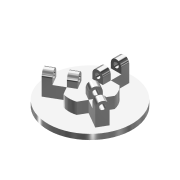
# Autodesk Inventor part: Base_Dedao
Saved by Autodesk Inventor 2020 (Build 240168000, 168)
## iProperties
Created: 2021-04-01
Part Number: Base_Dedao
Material: Generic
Document SubType Name: Modeling
Designer: deox
Density: 1 g/cm^3
Appearance: Chrome - Polished
Author: deox
Autodesk Inventor part; units mm, degrees
ref_plane "YZ Plane" through (0, 0, 0) normal (1, 0, 0) x (0, 1, 0)
ref_plane "XZ Plane" through (0, 0, 0) normal (0, 1, 0) x (-1, 0, 0)
ref_plane "XY Plane" through (0, 0, 0) normal (0, 0, 1) x (1, 0, 0)
sketch "Sketch1" plane through (0, 0, 0) normal (0, 1, 0) x (-1, 0, 0)
  circle A0 centre (0, 0) radius 11
  dimension "d0" = 22
  constraints: 1 centre point, 1 coincident
  measures "d0" diameter of A0
extrude "Extrusion1" add sketch "Sketch1" along normal blind 1.4
sketch "Sketch2" plane through (0, 1.4, 0) normal (0, 1, 0) x (1, 0, 0)
  line L0 (-11.1515, 11.0791) -> (11.8145, 11.0791) construction
  line L1 (11.8145, 11.0791) -> (11.8145, -11.3383) construction
  line L2 (11.8145, -11.3383) -> (-11.1515, -11.3383) construction
  line L3 (-11.1515, -11.3383) -> (-11.1515, 11.0791) construction
  circle A0 centre (0, 0) radius 11 projected
  circle A1 centre (0, 0) radius 11 projected
  line L4 (0, 0) -> (0, 2.0078)
  line L5 (0, 2.0078) -> (1.375, 2.0078)
  line L6 (1.375, 2.0078) -> (1.375, 4.0678)
  line L7 (1.375, 4.0678) -> (0, 4.0678)
  line L8 (1.375, 4.0678) -> (1.375, 6.8478)
  line L9 (1.375, 6.8478) -> (1.375, 8.9078)
  line L10 (1.375, 8.9078) -> (-1.375, 8.9078)
  line L11 (-1.375, 8.9078) -> (-1.375, 2.0078)
  line L12 (-1.375, 2.0078) -> (0, 2.0078)
  line L13 (1.375, 4.1034) -> (3.6499, 4.1034)
  line L14 (0, 0) -> (13.4051, 0) construction
  line L15 (4.2411, -0.8609) -> (5.3786, 1.1092)
  arc A2 (5.3786, 1.1092) -> (3.6499, 4.1034) centre (-0.1977, -0.1141) ccw
  line L16 (0, 0) -> (4.7463, 2.7403)
  line L17 (-1.7388, -1.0039) -> (-2.4263, 0.1869)
  line L18 (-2.4263, 0.1869) -> (-4.2104, -0.8431)
  line L19 (-4.2104, -0.8431) -> (-6.6179, -2.2331)
  line L20 (-1.0513, -2.1947) -> (-1.7388, -1.0039)
  line L21 (-6.6179, -2.2331) -> (-8.4019, -3.2631)
  line L22 (-7.0269, -5.6447) -> (-1.0513, -2.1947)
  line L23 (-8.4019, -3.2631) -> (-7.0269, -5.6447)
  line L24 (-4.2104, -0.8431) -> (-3.5229, -2.0339)
  line L25 (-4.2411, -0.8609) -> (-5.3786, 1.1092)
  line L26 (0, 0) -> (-1.7388, -1.0039)
  arc A3 (-3.6499, 4.1034) -> (-5.3786, 1.1092) centre (0.1977, -0.1141) ccw
  line L27 (0, 0) -> (-4.7463, 2.7403)
  line L28 (-1.375, 4.1034) -> (-3.6499, 4.1034)
  line L29 (1.7388, -1.0039) -> (1.0513, -2.1947)
  line L30 (1.0513, -2.1947) -> (2.8354, -3.2247)
  line L31 (2.8354, -3.2247) -> (5.2429, -4.6147)
  line L32 (2.4263, 0.1869) -> (1.7388, -1.0039)
  line L33 (5.2429, -4.6147) -> (7.0269, -5.6447)
  line L34 (8.4019, -3.2631) -> (2.4263, 0.1869)
  line L35 (7.0269, -5.6447) -> (8.4019, -3.2631)
  line L36 (2.8354, -3.2247) -> (3.5229, -2.0339)
  line L37 (2.8661, -3.2425) -> (1.7287, -5.2126)
  line L38 (0, 0) -> (1.7388, -1.0039)
  arc A4 (-1.7287, -5.2126) -> (1.7287, -5.2126) centre (0, 0.2283) ccw
  line L39 (0, 0) -> (0, -5.4806)
  line L40 (-2.8661, -3.2425) -> (-1.7287, -5.2126)
  dimension "d38" = 1.375
  dimension "d39" = 2.06
  dimension "d40" = 2.78
  dimension "d41" = 2.06
  dimension "d42" = 2.75
  dimension "d49" = 360
  dimension "d56" = 2.0078
  constraints: 74 end point, 9 point on circle, 9 point on line, 6 perpendicular, 3 centre point, 2 coincident, 2 horizontal, 2 vertical, 91 other
  measures "d38" distance of L4.end L5.end
  measures "d39" distance of L5.end L6.end
  measures "d40" distance of L6.end L8.end
  measures "d41" distance of L8.end L9.end
  measures "d42" distance of L9.end L10.end
  measures "d56" distance of L4.start L4.end
extrude "Extrusion2" add sketch "Sketch2" along normal blind 3 contours L27 A3 L28 L11 L12 L4 | L4 L5 L6 L8 L13 A2 L16 | L39 A4 L40 L22 L20 L26 | L26 L17 L18 L19 L25 A3 L27 | L16 A2 L15 L34 L32 L38 | L38 L29 L30 L31 L37 A4 L39 | L12 L11 L10 L9 L8 L6 L5 | L20 L22 L23 L21 L19 L18 L17 | L32 L34 L35 L33 L31 L30 L29
sketch "Sketch3" plane through (0, 4.4, 0) normal (0, 1, 0) x (1, 0, 0)
  line L0 (0, 0) -> (0, 2.0078)
  line L1 (0, 2.0078) -> (1.375, 2.0078)
  line L2 (1.375, 2.0078) -> (1.375, 4.0678)
  line L3 (1.375, 4.0678) -> (0, 4.0678)
  line L4 (0, 2.0078) -> (0, 4.0678)
  line L5 (1.375, 4.1034) -> (1.375, 8.9078) projected
  line L6 (1.375, 8.9078) -> (1.375, 6.8478)
  line L7 (1.375, 6.8478) -> (-1.375, 6.8478)
  line L8 (-1.375, 4.1034) -> (-1.375, 8.9078) projected
  line L9 (1.375, 8.9078) -> (-1.375, 8.9078) projected
  line L10 (-1.375, 6.8478) -> (-1.375, 8.9078)
  line L11 (-1.375, 8.9078) -> (1.375, 8.9078)
  line L12 (0, 2.0078) -> (-1.375, 2.0078)
  line L13 (-1.375, 2.0078) -> (-1.375, 4.0678)
  line L14 (-1.375, 4.0678) -> (0, 4.0678)
  line L15 (-1.7388, -1.0039) -> (-2.4263, 0.1869)
  line L16 (-2.4263, 0.1869) -> (-4.2104, -0.8431)
  line L17 (-4.2104, -0.8431) -> (-3.5229, -2.0339)
  line L18 (-1.7388, -1.0039) -> (-3.5229, -2.0339)
  line L19 (-1.7388, -1.0039) -> (-1.0513, -2.1947)
  line L20 (-1.0513, -2.1947) -> (-2.8354, -3.2247)
  line L21 (-2.8354, -3.2247) -> (-3.5229, -2.0339)
  line L22 (-8.4019, -3.2631) -> (-6.6179, -2.2331)
  line L23 (-6.6179, -2.2331) -> (-5.2429, -4.6147)
  line L24 (-5.2429, -4.6147) -> (-7.0269, -5.6447)
  line L25 (-7.0269, -5.6447) -> (-8.4019, -3.2631)
  line L26 (1.7388, -1.0039) -> (1.0513, -2.1947)
  line L27 (1.0513, -2.1947) -> (2.8354, -3.2247)
  line L28 (2.8354, -3.2247) -> (3.5229, -2.0339)
  line L29 (1.7388, -1.0039) -> (3.5229, -2.0339)
  line L30 (1.7388, -1.0039) -> (2.4263, 0.1869)
  line L31 (2.4263, 0.1869) -> (4.2104, -0.8431)
  line L32 (4.2104, -0.8431) -> (3.5229, -2.0339)
  line L33 (7.0269, -5.6447) -> (5.2429, -4.6147)
  line L34 (5.2429, -4.6147) -> (6.6179, -2.2331)
  line L35 (6.6179, -2.2331) -> (8.4019, -3.2631)
  line L36 (8.4019, -3.2631) -> (7.0269, -5.6447)
  point P0 (-4.2411, -0.8609)
  point P1 (-2.8661, -3.2425)
  point P2 (2.8661, -3.2425)
  point P3 (4.2411, -0.8609)
  dimension "d57" = 2.0078
  dimension "d58" = 1.375
  dimension "d59" = 2.06
  dimension "d60" = 2.06
  dimension "d63" = 360
  constraints: 68 end point, 5 perpendicular, 3 point on line, 3 vertical, 2 symmetric about line, 70 other
  measures "d57" distance of L0.start L0.end
  measures "d58" distance of L0.end L1.end
  measures "d59" distance of L1.end L2.end
  measures "d60" distance of L5.end L6.end
extrude "Extrusion3" add sketch "Sketch3" along normal blind 1.4
sketch "Sketch4" plane through (1.375, 1.4, -8.9078) normal (0, 0, -1) x (-1, 0, 0)
  line L0 (2.75, 4.4) -> (0, 4.4) projected
  circle A0 centre (1.375, 4.4) radius 1.375
  point P0 (1.375, -1.4)
  constraints: 1 midpoint, 3 other
extrude "Extrusion4" add sketch "Sketch4" against normal up to surface (2.06 mm away) contours L0 A0 picked at (1.7181, 4.7039)
pattern_circular "Circular Pattern1" count 3 over 360 about axis through (0, -10, 0) along (0, 1, 0) of "Extrusion4"
sketch "Sketch5" plane through (1.375, 4.4, -4.0678) normal (0, 0, -1) x (-1, 0, 0)
  line L0 (2.75, 1.4) -> (0, 1.4) projected
  circle A0 centre (1.375, 1.4) radius 1.375
  point P0 (1.375, -4.4)
  point P1 (0, 1.4)
  constraints: 1 midpoint, 3 other
extrude "Extrusion5" add sketch "Sketch5" against normal up to surface (2.06 mm away) contours L0 A0 picked at (1.7181, 1.7039)
pattern_circular "Circular Pattern2" count 3 over 360 about axis through (0, -10, 0) along (0, 1, 0) of "Extrusion5"
sketch "Sketch6" plane through (1.375, 1.4, -8.9078) normal (0, 0, -1) x (-1, 0, 0)
  line L0 (0, 0) -> (0, 4.4) projected
  line L1 (2.75, 0) -> (2.75, 4.4) projected
  line L2 (0, 4.4) -> (2.75, 4.4)
  circle A0 centre (1.375, 4.4) radius 0.6874
  point P0 (1.375, -1.4)
  dimension "d77" = 1.3749
  constraints: 2 end point, 1 centre point, 1 horizontal, 1 midpoint
  measures "d77" diameter of A0
extrude "Extrusion6" cut sketch "Sketch6" against normal up to surface (6.9 mm away)
pattern_circular "Circular Pattern3" count 3 over 360 about axis through (0, -10, 0) along (0, 1, 0) of "Extrusion6"
body "Solid1"
